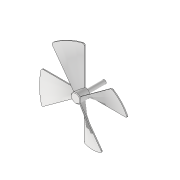
# Autodesk Inventor part: Ruehrwerk
Saved by Autodesk Inventor 2020 (Build 240168000, 168)
## iProperties
Created: 2020-04-08
Part Number: Ruehrwerk
Material: Generisch
Document SubType Name: Modeling
Designer: franz
Density: 1 g/cm^3
Appearance: Vorgabe
Author: franz
Autodesk Inventor part; units mm, degrees
ref_plane "YZ Plane" through (0, 0, 0) normal (1, 0, 0) x (0, 1, 0)
ref_plane "XZ Plane" through (0, 0, 0) normal (0, 1, 0) x (-1, 0, 0)
ref_plane "XY Plane" through (0, 0, 0) normal (0, 0, 1) x (1, 0, 0)
sketch "Skizze1" plane through (0, 0, 0) normal (0, 0, 1) x (1, 0, 0)
  circle A0 centre (0, 0) radius 25
  dimension "d0" = 50
  constraints: 1 centre point, 1 coincident
  measures "d0" diameter of A0
extrude "Extrusion1" add sketch "Skizze1" along normal blind 50
sketch "Skizze2" plane through (0, 0, 0) normal (0, 0, -1) x (-1, 0, 0)
  circle A0 centre (0, 0) radius 10
  dimension "d3" = 20
  constraints: 1 centre point, 1 coincident
  measures "d3" diameter of A0
extrude "Extrusion2" add sketch "Skizze2" along normal blind 150
sketch "Skizze3" plane through (0, 0, 0) normal (0, 1, 0) x (-1, 0, 0)
  line L0 (-25, 0) -> (-25, 50) projected
  line L1 (-25, 5) -> (-225, 5)
  line L2 (-225, 5) -> (-225, 0)
  line L3 (-225, 0) -> (-25, 0)
  line L4 (-25, 0) -> (-25, 5)
  line L5 (25, 0) -> (-25, 0) projected
  point P0 (0, 0)
  dimension "d6" = 200
  dimension "d7" = 5
  dimension "d8" = 50
  dimension "d18" = 0
  constraints: 8 end point, 2 parallel, 1 horizontal, 1 perpendicular, 1 point on line
  measures "d6" distance of L3.end L2.end
  measures "d7" distance of L2.end L1.end
  measures "d8" distance of L0.end L0.start
  measures "d18" distance between parallel lines of L5 L3
coil "Spirale1" sketch "Skizze3" operation add axis through (0, 0, -10) along (0, 0, 1) pitch 400 turns 0.1 hand right
fillet "Rundung1" radius 8 2 edges at (225, 0, 2.5) (182.0288, 132.2517, 42.5)
pattern_circular "Runde Anordnung1" count 4 over 360 about axis through (0, 0, -10) along (0, 0, 1) of "Spirale1", "Rundung1"
chamfer "Fase1" distance 3 angle 45 1 edges at (-25, 0, 50)
